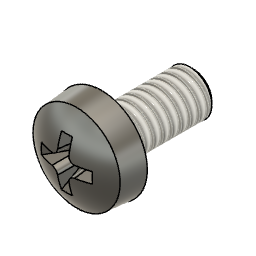
6bdba332-45ad-4538-b0bd-f7503bdef819 (Autodesk Fusion 360 design; units mm, degrees)
description: Raised Cheese Head Screw DIN 7985 - M2 x 4 - H
Autodesk Fusion 360 part; units mm, degrees
sketch "Sketch1" plane through (0, 0, 0) normal (0, 1, 0) x (1, 0, 0)
  line L0 (-1, 4) -> (0, 4)
  line L1 (0, 4) -> (0, -1.72)
  line L2 (-0.9, 0) -> (-2, 0)
  line L3 (-2, 0) -> (-1.9045, -1.0916)
  arc A0 (-1.9045, -1.0916) -> (0, -1.72) centre (0, 1.48) ccw
  line L4 (-0.9, 0) -> (-0.9, 0.64)
  line L5 (-0.9, 0.64) -> (-1, 0.64)
  line L6 (-1, 0.64) -> (-1, 4)
  dimension "d66" = 4
  dimension "d67" = 1.72
  dimension "d68" = 4
  dimension "d70" = 3.2
  dimension "d79" = 2
  dimension "d81" = 1.8
  dimension "d84" = 0.64
  dimension "d85" = 85
  constraint collinear origin L1.end L0.end
  constraint coincident origin L2
  constraint vertical L1
  constraint coincident L1 A0.centre
  constraint perpendicular L2 L4
  constraint perpendicular L4 L5
  constraint perpendicular L0 L6
  constraint coincident L0.start L6.end
  constraint vertical L6
  constraint vertical L4
  measures "d67" vertical distance of L1.end L2.end
  measures "d68" distance of origin L0.end
  measures "d70" radius of A0
  measures "d84" distance of L2 L5
  measures "d85" angle of L2 L3
revolve "Revolve1" add sketch "Sketch1" angle 360 about axis through (0, 0, -4) along (0, 0, 1) makes body 1
ref_plane "WorkPlane1" through (0, 0, 1.72) normal (0, 0, 1) x (1, 0, 0)
sketch "Sketch2" plane through (0, 0, 1.72) normal (0, 0, 1) x (1, 0, 0)
  line L0 (-0.25, 1.25) -> (-0.25, 0.25)
  line L1 (-0.25, 0.25) -> (-1.25, 0.25)
  line L2 (0, 0) -> (0, 1.25) construction
  line L3 (0.25, 0.25) -> (1.25, 0.25)
  line L4 (0.25, 1.25) -> (0.25, 0.25)
  line L5 (0.25, -0.25) -> (1.25, -0.25)
  line L6 (0.25, -1.25) -> (0.25, -0.25)
  line L7 (-0.25, -1.25) -> (-0.25, -0.25)
  line L8 (-0.25, -0.25) -> (-1.25, -0.25)
  line L9 (-0.25, 1.25) -> (0.25, 1.25)
  line L10 (-1.25, 0.25) -> (-1.25, -0.25)
  line L11 (-0.25, -1.25) -> (0.25, -1.25)
  line L12 (1.25, -0.25) -> (1.25, 0.25)
  line L13 (-1.25, 0) -> (1.25, 0) construction
  dimension "d22" = 0.5
  dimension "d57" = 2.5
  dimension "d99" = 2.5
  constraint perpendicular L0 L1
  constraint symmetric L0.start L2 L4.start
  constraint symmetric L0.end L2 L3.start
  constraint symmetric L1.end L2 L3.end
  constraint perpendicular L4 L9
  constraint perpendicular L8 L10
  constraint equal L9 L10
  constraint equal L0 L1
  constraint horizontal L0.start L2.end
  constraint vertical L2
  constraint collinear L4 L6
  constraint midpoint L10 L13.start
  constraint midpoint L12 L13.end
  constraint perpendicular L12 L13
  constraint coincident L2.start L13
  constraint horizontal L8
  constraint horizontal L5
  constraint horizontal L11
  constraint coincident origin L2
  measures "d22" horizontal distance of L0.start L4.start
  measures "d57" distance of L10 L12
  measures "d99" distance of L9 L11
extrude "Extrude1" add sketch "Sketch2" against normal blind 1 draft -4 separate body makes body 2
draft "Draft1" angle -30 neutral plane through (0, 0, 1.72) pull (0, 0, 1) 4 faces at (1.2267, 0.06, 1.3867) (-0.06, 1.2267, 1.3867) (-1.2267, 0.06, 1.3867) (0.06, -1.2267, 1.3867) on bodies 2
fillet "Fillet3" radius 0.25 4 edges at (-0.215, 0.215, 1.22) (0.215, 0.215, 1.22) (0.215, -0.215, 1.22) (-0.215, -0.215, 1.22) on bodies 2
combine "Combine1" operation cut target body 1 tool bodies 2
thread "Thread2" "ISO Metric profile 2.0 M2x0.4 6g" major diameter 1.9335 minor diameter 1.478 pitch 0.4 angle 60 resizes the face on face at (-0.995, 0.0996, -2.88) on bodies 1
sketch "Sketch5" plane through (0, 0, 0) normal (0, 1, 0) x (1, 0, 0)
  line L0 (0, 4) -> (0, -1.72)
  line L1 (0, 4) -> (-1.02, 4)
  line L2 (-1.02, 4) -> (-1.02, 3.8)
  line L3 (-1.02, 3.8) -> (-0.82, 4)
  dimension "d93" = 45
  dimension "d94" = 0.82
  dimension "d95" = 1.02
  constraint coincident L0.start L1.start
  constraint perpendicular L0 L1
  constraint perpendicular L1 L2
  constraint coincident L1 L3.end
  measures "d93" angle of L2 L3
  measures "d94" horizontal distance of origin L3.end
  measures "d95" horizontal distance of origin L1.end
revolve "Revolve2" cut sketch "Sketch5" angle 360 about axis through (0, 0, 1.75) along (0, 0, 1) bodies 1
equation "adsk_nomlen = 4.00 mm"
equation "adsk_headh = 1.72 mm"
equation "adsk_headdia = 4.00 mm"
equation "adsk_nomdia = 2.00 mm"
equation "d22 = adsk_philwidth"
equation "adsk_phildia = 2.50 mm"
equation "d31 = -adsk_phildepth"
equation "adsk_phildepth = 1.00 mm"
equation "d57 = adsk_phildia"
equation "d59 = adsk_phildia * 0.1"
equation "d66 = adsk_headdia"
equation "d67 = adsk_headh"
equation "d68 = adsk_nomlen"
equation "d70 = adsk_headdia * 0.8"
equation "d71 = adsk_headh"
equation "adsk_thrlen = 3.36 mm"
equation "d79 = adsk_nomdia"
equation "d81 = adsk_nomdia - ( adsk_pitch1 / 2 )"
equation "adsk_pitch1 = 0.40 mm"
equation "d84 = adsk_nomlen - adsk_thrlen"
equation "d94 = d95 - ( adsk_pitch1 / 2 )"
equation "d95 = adsk_nomdia * 0.51"
equation "adsk_philwidth = adsk_phildia / 5"
equation "d99 = adsk_phildia"
